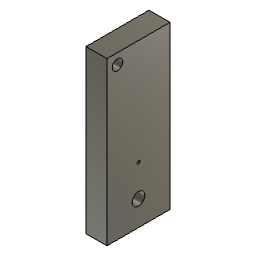
ensamble_pata (Autodesk Fusion 360 archive; units mm, degrees)
design "pierna"
Autodesk Fusion 360 part; units mm, degrees
sketch "Sketch1" plane through (0, 0, 0) normal (1, 0, 0) x (0, 1, 0)
  line L0 (0, 0) -> (30, 0)
  line L1 (30, 0) -> (30, 77.1664)
  line L2 (30, 77.1664) -> (0, 77.1664)
  line L3 (0, 77.1664) -> (0, 0)
  dimension "d1" = 30
  constraint horizontal L0
  constraint vertical L1
  constraint horizontal L2
  constraint vertical L3
  constraint coincident L0.start L3.end
  measures "d1" distance of L0.start L0.end
extrude "Extrude1" add sketch "Sketch1" along normal blind 10
sketch "Sketch2" plane through (10, 0, 0) normal (1, 0, 0) x (0, 1, 0)
  line L0 (0, 77.1664) -> (0, 0)
  line L1 (0, 0) -> (30, 0)
  line L2 (30, 0) -> (30, 77.1664)
  line L3 (30, 77.1664) -> (0, 77.1664)
  point P0 (15, 11.8696)
  point P1 (15, 26.8696)
  dimension "d7" = 15
  measures "d7" distance of P0 P1
hole "Hole1" at (10, 15, 11.8696) direction (-1, 0, 0) diameter 6 depth 30 tip angle 118
hole "Hole2" at (10, 15, 26.8696) direction (-1, 0, 0) diameter 1.5 depth 3 tip angle 118
sketch "Sketch3" plane through (10, 0, 0) normal (1, 0, 0) x (0, 1, 0)
  circle A0 centre (15, 26.8696) radius 0.75
  circle A1 centre (15, 11.8696) radius 3
  line L0 (0, 77.1664) -> (0, 0)
  line L1 (0, 0) -> (30, 0)
  line L2 (30, 0) -> (30, 77.1664)
  line L3 (30, 77.1664) -> (0, 77.1664)
  circle A2 centre (5, 72.1664) radius 2.5
  dimension "d11" = 5
  dimension "d12" = 5
  dimension "d13" = 5
  measures "d11" diameter of A2
  measures "d12" distance of L3 A2.centre
  measures "d13" distance of L0 A2.centre
extrude "Extrude2" cut sketch "Sketch3" against normal blind 16 contours A2
